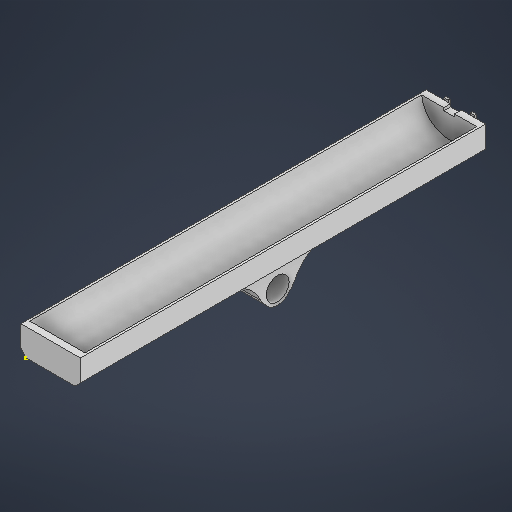
# Autodesk Inventor part: profilrampa
Saved by Autodesk Inventor 2026.2 (Build 302298000, 298)
## iProperties
Created: 2025-11-25
Part Number: profilrampa
Material: Generic
Document SubType Name: Modeling
Designer: janek
Density: 1 g/cm^3
Appearance: Default
Author: janek
Autodesk Inventor part; units mm, degrees
ref_plane "YZ Plane" through (0, 0, 0) normal (1, 0, 0) x (0, 1, 0)
ref_plane "XZ Plane" through (0, 0, 0) normal (0, 1, 0) x (-1, 0, 0)
ref_plane "XY Plane" through (0, 0, 0) normal (0, 0, 1) x (1, 0, 0)
sketch "Sketch1" plane through (0, 0, 0) normal (0, 1, 0) x (-1, 0, 0)
  line L0 (0, 0) -> (44, 0)
  line L1 (44, 0) -> (44, -300)
  line L2 (44, -300) -> (0, -300)
  line L3 (0, -300) -> (0, 0)
  dimension "d0" = 300
  dimension "d1" = 44
  constraints: 8 end point, 2 parallel, 1 horizontal, 1 perpendicular
  measures "d0" distance of L0.end L1.end
  measures "d1" distance between parallel lines of L3 L1
extrude "Extrusion1" add sketch "Sketch1" along normal blind 20
sketch "Sketch2" plane through (-44, 0, 0) normal (0, 0, 1) x (1, 0, 0)
  line L0 (44, 20) -> (0, 20) projected
  line L1 (44, 0) -> (0, 0) projected
  line L2 (0, 0) -> (44, 0)
  line L3 (44, 0) -> (44, 22)
  line L4 (44, 22) -> (0, 22)
  line L5 (0, 22) -> (0, 0)
  circle A0 centre (22, 22) radius 20.5
  dimension "d17" = 22
  dimension "d18" = 41
  dimension "d19" = 22
  constraints: 8 end point, 2 parallel, 1 centre point, 1 horizontal, 1 midpoint, 1 perpendicular
  measures "d17" distance of L2.end L3.end
  measures "d18" diameter of A0
  measures "d19" distance from line of L5 A0.centre
extrude "Extrusion2" cut sketch "Sketch2" against normal up to surface (300 mm away) contours A0 L0 | L0 A0 L4 | L4 A0
sketch "Sketch3" plane through (-44, 0, 0) normal (0, 0, 1) x (1, 0, 0)
  line L0 (0, 0) -> (0, 20) projected
  line L1 (0, 20) -> (44, 20)
  line L2 (44, 20) -> (44, 0)
  line L3 (44, 0) -> (0, 0)
  line L4 (0, 0) -> (0, 20)
  constraints: 8 end point, 2 parallel, 1 horizontal, 1 perpendicular
extrude "Extrusion3" add sketch "Sketch3" against normal blind 5
sketch "Sketch4" plane through (0, 0, -300) normal (0, 0, -1) x (-1, 0, 0)
  line L0 (0, 0) -> (0, 20) projected
  line L1 (44, 0) -> (0, 0) projected
  line L2 (0, 20) -> (44, 20)
  line L3 (44, 20) -> (44, 0)
  line L4 (44, 0) -> (0, 0)
  line L5 (0, 0) -> (0, 20)
  constraints: 8 end point, 2 parallel, 1 horizontal, 1 perpendicular
extrude "Extrusion4" add sketch "Sketch4" against normal blind 5
chamfer "Chamfer1" distance 4 angle 45 1 edges at (0, 0, -150)
chamfer "Chamfer2" distance 4 angle 45 1 edges at (-44, 0, -150)
sketch "Sketch5" plane through (0, 20, -300) normal (0, 0, -1) x (-1, 0, 0)
  line L0 (0, 0) -> (44, 0)
  line L1 (44, 0) -> (44, -20)
  line L2 (44, -20) -> (0, -20)
  line L3 (0, -20) -> (0, 0)
  line L4 (44, -16) -> (40, -20) projected
  line L5 (4, -20) -> (0, -16) projected
  line L6 (22, 0) -> (22, -20)
  line L7 (0, -10) -> (44, -10)
  line L8 (11.8539, 0) -> (11.8539, -20)
  line L9 (32.3539, 0) -> (32.3539, -20)
  line L10 (10.8539, 0) -> (10.8539, -20)
  line L11 (33.3539, 0) -> (33.3539, -20)
  line L12 (0, -9) -> (44, -9)
  circle A0 centre (11.8539, 0) radius 2
  circle A1 centre (32.3539, 0) radius 2
  point P0 (0, -20)
  point P1 (2, -18)
  point P2 (42, -18)
  point P3 (11.8539, -2)
  point P4 (10.8539, -1.7321)
  point P5 (10.8539, -10)
  point P6 (33.3539, -10)
  point P7 (33.3539, -1.7321)
  point P8 (32.3539, -2)
  point P9 (32.3539, -9)
  point P10 (11.8539, -9)
  dimension "d20" = 20
  dimension "d21" = 44
  dimension "d23" = 2
  dimension "d24" = 2
  dimension "d25" = 20.5
  dimension "d26" = 11.8539
  dimension "d27" = 1
  dimension "d28" = 1
  dimension "d29" = 9
  dimension "d30" = 4
  dimension "d31" = 4
  constraints: 20 end point, 6 point on line, 5 midpoint, 4 vertical, 2 centre point, 2 coincident, 2 horizontal, 2 perpendicular, 1 parallel, 8 other
  measures "d20" distance of L3.start L0.start
  measures "d21" distance between parallel lines of L1 L3
  measures "d23" horizontal distance of L3.start point (2, -18)
  measures "d24" horizontal distance of L1.end point (42, -18)
  measures "d25" distance between parallel lines of L9 L8
  measures "d26" distance between parallel lines of L3 L8
  measures "d27" distance between parallel lines of L10 L8
  measures "d28" distance between parallel lines of L9 L11
  measures "d29" distance between parallel lines of L12 L0
  measures "d30" diameter of A0
  measures "d31" diameter of A1
extrude "Extrusion5" add sketch "Sketch5" along normal blind 2.5 contours A0 L8 L12 L10 | L12 L8 L7 L10 | L12 L6 L7 L8 | L12 L9 L7 L6 | A1 L11 L12 L9 | L12 L11 L7 L9
sketch "Sketch7" plane through (-33.3539, 10, -300) normal (0, -1, 0) x (1, 0, 0)
  line L0 (22.5, -2.5) -> (0, -2.5)
  line L1 (0, -2.5) -> (0, -4)
  line L2 (0, -4) -> (22.5, -4)
  line L3 (22.5, -4) -> (22.5, -2.5)
  line L4 (0, 0) -> (0, -2.5) projected
  line L5 (22.5, -4) -> (21.5, -4)
  line L6 (21.5, -2.5) -> (22.5, -2.5)
  line L7 (22.5, -2.5) -> (22.5, -4)
  line L8 (21.5, 0) -> (21.5, -2.5) projected
  line L9 (3, -2.5) -> (0, -2.5)
  line L10 (0, -2.5) -> (0, -4)
  line L11 (0, -4) -> (3, -4)
  line L12 (3, -4) -> (3, -2.5)
  line L13 (22.5, -2.5) -> (0, -2.5) projected
  line L14 (22.5, -4) -> (19.5, -4)
  line L15 (19.5, -4) -> (19.5, -2.5)
  line L16 (19.5, -2.5) -> (22.5, -2.5)
  line L17 (22.5, -2.5) -> (22.5, -4)
  point P0 (33.3539, 300)
  point P1 (22.5, -3.25)
  point P2 (19.5, -4)
  point P3 (19.5, -2.5)
  point P4 (3, -4)
  dimension "d36" = 1.5
  dimension "d37" = 3
  dimension "d38" = 3
  constraints: 30 end point, 8 parallel, 4 horizontal, 3 perpendicular, 2 point on line, 1 collinear, 1 midpoint, 2 other
  measures "d36" distance between parallel lines of L0 L2
  measures "d37" distance from line of point (22.5, -3.25) L15
  measures "d38" distance between parallel lines of L12 L1
extrude "Extrusion6" add sketch "Sketch7" against normal blind 3 contours L15 L2 L12 L0
extrude "Extrusion7" add sketch "Sketch7" against normal blind 9 contours L3 L2 L15 L0 | L12 L2 L1 L0
sketch "Sketch8" plane through (0, 0, 0) normal (0, -1, 0) x (1, 0, 0)
  line L0 (-44, -300) -> (-40, -300) projected
  line L1 (-40, -300) -> (-35, -300)
  line L2 (-35, -300) -> (-35, -290)
  line L3 (-35, -290) -> (-40, -290)
  line L4 (-40, -290) -> (-40, -300)
  line L5 (-4, 0) -> (-4, -300) projected
  point P0 (0, 0)
  point P1 (-37.5, -290)
  dimension "d43" = 10
  dimension "d44" = 5
  constraints: 8 end point, 2 parallel, 1 horizontal, 1 midpoint, 1 perpendicular
  measures "d43" distance from line of point (-37.5, -290) L1
  measures "d44" distance between parallel lines of L2 L4
extrude "Extrusion8" add sketch "Sketch8" along normal blind 6
sketch "Sketch9" plane through (-40, -6, -300) normal (-1, 0, 0) x (0, 0, 1)
  point P0 (300, 6)
  point P1 (5.0353, 2.5819)
hole "Hole1" at (-40, -3.4181, -294.9647) direction (1, 0, 0) diameter 3.5 end through all
sketch "Sketch10" plane through (-40, -6, -300) normal (-1, 0, 0) x (0, 0, 1)
  line L0 (10, 6) -> (0, 6) projected
  line L1 (0, 0) -> (10, 0) projected
  arc A0 (10, 6) -> (7.7341, 0) centre (16.1486, 0.2502) ccw
  arc A1 (5, 0) -> (8.2733, 3.2242) centre (4.0632, 4.2247) ccw
  line L2 (0, 6) -> (0, 0) projected
  arc A2 (2.2659, 0) -> (0, 6) centre (-6.1486, 0.2502) ccw
  arc A3 (1.7267, 3.2242) -> (5, 0) centre (5.9368, 4.2247) ccw
  line L3 (10, 6) -> (10, 0) projected
  point P0 (300, 6)
  point P1 (1.7267, 3.2242)
  point P2 (8.0453, 2.531)
  dimension "d54" = 8.4182
  dimension "d55" = 8.4182
  dimension "d56" = 4.3273
  dimension "d57" = 4.3273
  dimension "d58" = 2.2659
  dimension "d59" = 2.2659
  dimension "d60" = 5.9368
  dimension "d61" = 3.2242
  dimension "d64" = 1.7267
  constraints: 10 point on circle, 4 centre point, 1 midpoint, 1 point on line
  measures "d54" radius of A0
  measures "d55" radius of A2
  measures "d56" radius of A3
  measures "d57" radius of A1
  measures "d58" distance of L1.end A0.end
  measures "d59" distance of A2.start L1.start
  measures "d60" distance from line of L2 A3.centre
  measures "d61" vertical distance of point (1.727, 3.224) A2.start
  measures "d64" distance from line of L3 A1.end
extrude "Extrusion10" cut sketch "Sketch10" against normal blind 6 contours L3 L1 A0 A1 | A2 A3 L1 L2 | A0 L1 A1 | A2 A3 L1
fillet "Fillet1" radius 2 1 edges at (-37.5, -6, -295)
sketch "Sketch11" plane through (0, 0, 0) normal (0, -1, 0) x (1, 0, 0)
  line L0 (-40, -290) -> (-40, 0) projected
  line L1 (-4, 0) -> (-4, -300) projected
  line L2 (-40, -175) -> (-4, -175)
  line L3 (-4, -175) -> (-4, -125)
  line L4 (-4, -125) -> (-40, -125)
  line L5 (-40, -125) -> (-40, -175)
  line L6 (-40, 0) -> (-4, 0) projected
  line L7 (-4, -300) -> (-35, -300) projected
  point P0 (0, 0)
  point P1 (-4, -175)
  dimension "d68" = 125
  dimension "d69" = 125
  constraints: 8 end point, 2 parallel, 2 point on line, 1 horizontal, 1 perpendicular
  measures "d68" distance between parallel lines of L6 L4
  measures "d69" distance between parallel lines of L2 L7
extrude "Extrusion11" add sketch "Sketch11" along normal blind 25 contours L0 L4 L1 L2
sketch "Sketch12" plane through (-40, -25, -175) normal (-1, 0, 0) x (0, 0, 1)
  point P0 (175, 25)
sketch "Sketch13" plane through (-40, -25, -175) normal (-1, 0, 0) x (0, 0, 1)
  line L0 (0, 25) -> (50, 25) projected
  line L1 (15, 25) -> (15, -0.135)
  line L2 (35, 25) -> (35, -0.135)
  line L3 (0, 25) -> (0, 0) projected
  line L4 (50, 25) -> (50, 0) projected
  arc A0 (50, 25) -> (35, -0.135) centre (64.9879, -0.9878) ccw
  line L5 (50, 0) -> (0, 0) projected
  arc A1 (25, 0) -> (39.2265, 14.386) centre (12.7885, 26.3036) ccw
  line L6 (25, 25) -> (25, 0)
  arc A2 (15, -0.135) -> (0, 25) centre (-14.9879, -0.9878) ccw
  arc A3 (10.7735, 14.386) -> (25, 0) centre (37.2115, 26.3036) ccw
  circle A4 centre (25, 12.5) radius 8.5
  arc A5 (16.5915, 5.9121) -> (33.4085, 5.9121) centre (25, 12.5) ccw
  point P0 (175, 25)
  point P1 (35, 0)
  point P2 (35.0041, 0)
  point P3 (37.6622, 11.3939)
  point P4 (12.3378, 11.3939)
  dimension "d73" = 15
  dimension "d74" = 15
  dimension "d75" = 29
  dimension "d76" = 30
  dimension "d77" = 14.386
  dimension "d78" = 17
  constraints: 13 point on circle, 6 centre point, 6 end point, 3 midpoint, 3 symmetric about line, 3 vertical, 2 point on line, 1 concentric, 2 other
  measures "d73" distance between parallel lines of L3 L1
  measures "d74" distance between parallel lines of L4 L2
  measures "d75" radius of A1
  measures "d76" radius of A0
  measures "d77" distance from line of L5 A1.end
  measures "d78" diameter of A4
extrude "Extrusion12" cut sketch "Sketch13" against normal through all contours A2 A3 L5 L3 | A2 A3 | A3 A5 L5 L1 | L1 A2 A3 | A4 L6 | L6 A4 | A1 A5 L2 L5 | L6 A5 A1 | A3 A5 L6 | L4 L5 A0 A1 | A1 A0 L2 | A1 A0
sketch "Sketch14" plane through (0, 20, -300) normal (0, 0, -1) x (-1, 0, 0)
  line L0 (1.5978, 0) -> (42.4022, 0) projected
  line L1 (18, 0) -> (26, 0)
  line L2 (26, 0) -> (26, -2)
  line L3 (26, -2) -> (18, -2)
  line L4 (18, -2) -> (18, 0)
  line L5 (0, -16) -> (0, 0) projected
  line L6 (44, -16) -> (44, 0) projected
  point P0 (0, -20)
  point P1 (18, -1)
  point P2 (26, 0)
  dimension "d81" = 18
  dimension "d82" = 18
  dimension "d83" = 2
  constraints: 8 end point, 2 parallel, 1 horizontal, 1 midpoint, 1 perpendicular, 1 point on line
  measures "d81" distance from line of L5 point (18, -1)
  measures "d82" distance from line of L6 L2.end
  measures "d83" distance between parallel lines of L0 L3
extrude "Extrusion13" cut sketch "Sketch14" against normal blind 10
body "Solid1"
